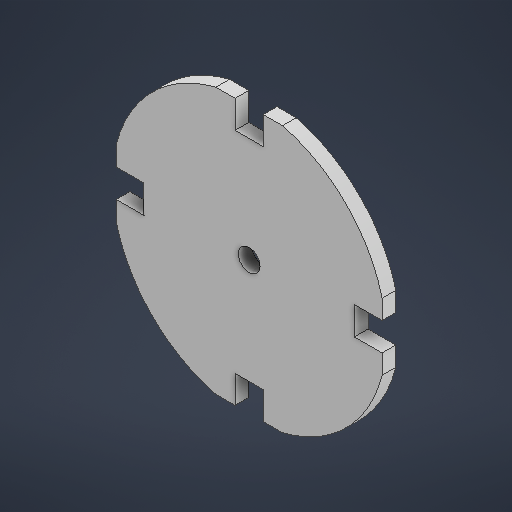
# Autodesk Inventor part: plate_lower
Saved by Autodesk Inventor 2027 (Build 310192000, 192)
## iProperties
Created: 2026-10-07
Part Number: plate_lower
Material: Generisch
Document SubType Name: Modeling
Designer: luca
Density: 1 g/cm^3
Appearance: Vorgabe
Author: luca
Autodesk Inventor part; units mm, degrees
ref_plane "YZ Plane" through (0, 0, 0) normal (1, 0, 0) x (0, 1, 0)
ref_plane "XZ Plane" through (0, 0, 0) normal (0, 1, 0) x (-1, 0, 0)
ref_plane "XY Plane" through (0, 0, 0) normal (0, 0, 1) x (1, 0, 0)
sketch "Skizze1" plane through (0, 0, 0) normal (0, 1, 0) x (-1, 0, 0)
  circle A0 centre (0, 0) radius 100
  dimension "d0" = 200
  constraints: 1 centre point, 1 coincident
  measures "d0" diameter of A0
extrude "Extrusion1" add sketch "Skizze1" along normal blind 10
sketch "Skizze2" plane through (0, 10, 0) normal (0, 1, 0) x (1, 0, 0)
  circle A0 centre (0, 0) radius 100 projected
  circle A1 centre (-87, 0) radius 3.1
  dimension "d3" = 6.2
  dimension "d4" = 87
  dimension "d5" = 200
  constraints: 1 centre point, 1 horizontal alignment
  measures "d3" diameter of A1
  measures "d4" distance of A1.centre A0.centre
  measures "d5" diameter of A0
extrude "Extrusion2" cut sketch "Skizze2" against normal through all contours A1
chamfer "Fasen1" distance 3 angle 45 1 edges at (-90.1, 0, 0)
sketch "Skizze3" plane through (0, 10, 0) normal (0, 1, 0) x (1, 0, 0)
  circle A0 centre (-87, 0) radius 3.1 projected
  circle A1 centre (0, 0) radius 100 projected
  line L0 (-97, -24.3105) -> (-97, 24.3105)
  circle A2 centre (0, 0) radius 100 projected
  point P0 (-97, -24.3105)
  dimension "d11" = 10
  constraints: 2 end point, 1 point on circle, 1 vertical, 2 other
  measures "d11" distance from line of A0.centre L0
extrude "Extrusion3" cut sketch "Skizze3" against normal through all contours L0 A1 picked at (-97.7491, 4.0825)
pattern_circular "Runde Anordnung3" count 4 over 360 about axis through (0, -10, 0) along (0, 1, 0) of "Extrusion2", "Fasen1"
pattern_circular "Runde Anordnung4" count 4 over 360 about axis through (0, -10, 0) along (0, 1, 0) of "Extrusion3"
sketch "Skizze4" plane through (0, 0, 0) normal (0, -1, 0) x (1, 0, 0)
  circle A0 centre (0, 0) radius 8
  dimension "d26" = 16
  constraints: 1 centre point, 1 coincident
  measures "d26" diameter of A0
extrude "Extrusion4" cut sketch "Skizze4" against normal through all
sketch "Skizze5" plane through (0, 0, 0) normal (0, -1, 0) x (1, 0, 0)
  circle A0 centre (0, 0) radius 8 projected
  circle A1 centre (0, -87) radius 6.1 projected
  circle A2 centre (0, 87) radius 6.1 projected
  line L0 (-24.3105, -97) -> (24.3105, -97) projected
  arc A3 (24.3105, -97) -> (97, -24.3105) centre (0, 0) ccw projected
  line L1 (97, -24.3105) -> (97, 24.3105) projected
  arc A4 (97, 24.3105) -> (24.3105, 97) centre (0, 0) ccw projected
  line L2 (24.3105, 97) -> (-24.3105, 97) projected
  arc A5 (-24.3105, 97) -> (-97, 24.3105) centre (0, 0) ccw projected
  line L3 (-97, 24.3105) -> (-97, -24.3105) projected
  arc A6 (-97, -24.3105) -> (-24.3105, -97) centre (0, 0) ccw projected
  circle A7 centre (-87, 0) radius 6.1 projected
  circle A8 centre (87, 0) radius 6.1 projected
  line L4 (-10.25, 76.75) -> (10.25, 76.75)
  line L5 (10.25, 76.75) -> (10.25, 97.25)
  line L6 (10.25, 97.25) -> (-10.25, 97.25)
  line L7 (-10.25, 97.25) -> (-10.25, 76.75)
  line L8 (-10.25, 76.75) -> (10.25, 97.25) construction
  line L9 (10.25, 76.75) -> (-10.25, 97.25) construction
  point P0 (10.25, 97)
  point P1 (-10.25, 97)
  dimension "d29" = 20.5
  dimension "d30" = 20.5
  constraints: 12 end point, 2 midpoint, 2 parallel, 1 horizontal, 1 perpendicular
  measures "d29" distance of L6.end L5.end
  measures "d30" distance of L5.end L4.end
extrude "Extrusion5" cut sketch "Skizze5" against normal through all contours A2 | L2 L5 L4 L7
pattern_circular "Runde Anordnung5" count 4 over 360 about axis through (0, 0, 0) along (0, 1, 0) of "Extrusion5"
